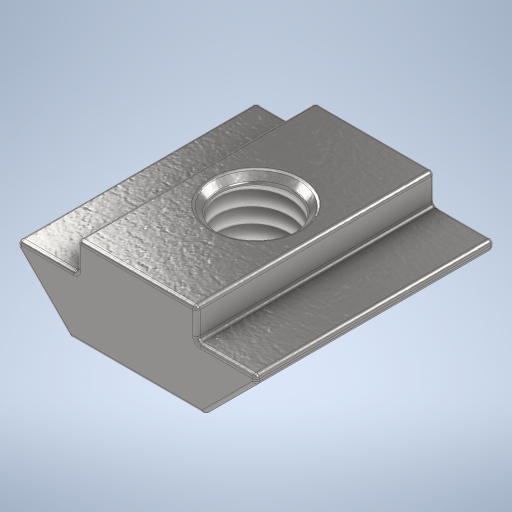
# Autodesk Inventor part: M6 T SLOT NUT 3030
Saved by Autodesk Inventor 2024 (Build 280153000, 153)
## iProperties
Created: 2024-12-02
Part Number: M6 T SLOT NUT 3030
Material: Steel, Galvanized
Document SubType Name: Modeling
Designer: Ishaan
Density: 7.85 g/cm^3
Appearance: Galvanized
Author: Ishaan
Autodesk Inventor part; units mm, degrees
ref_plane "YZ Plane" through (0, 0, 0) normal (1, 0, 0) x (0, 1, 0)
ref_plane "XZ Plane" through (0, 0, 0) normal (0, 1, 0) x (-1, 0, 0)
ref_plane "XY Plane" through (0, 0, 0) normal (0, 0, 1) x (1, 0, 0)
sketch "Sketch1" plane through (0, 0, 0) normal (0, 0, 1) x (1, 0, 0)
  line L0 (4, -3) -> (-4, -3)
  line L1 (-4, -3) -> (-4, 3)
  line L2 (-4, 3) -> (4, 3)
  line L3 (4, 3) -> (4, -3)
  line L4 (4, -3) -> (-4, 3) construction
  line L5 (-4, -3) -> (4, 3) construction
  line L6 (-8, 1) -> (8, 1)
  line L7 (8, 1) -> (8, -3)
  line L8 (8, -3) -> (-8, -3)
  line L9 (-8, -3) -> (-8, 1)
  point P0 (0, 0)
  point P1 (0, -3)
  point P2 (4, 1)
  point P3 (-4, 1)
  dimension "d0" = 2
  dimension "d1" = 4
  dimension "d2" = 16
  dimension "d3" = 8
  constraints: 20 end point, 4 midpoint, 4 parallel, 2 horizontal, 2 perpendicular
  measures "d0" distance between parallel lines of L2 L6
  measures "d1" distance of L8.end L6.start
  measures "d2" distance of L7.end L8.end
  measures "d3" distance of L1.end L2.end
extrude "Extrusion1" add sketch "Sketch1" along normal mid plane 16
chamfer "Chamfer1" distance 3.5 angle 45 2 edges at (-8, -3, 0) (8, -3, 0)
sketch "Sketch2" plane through (-4, 3, 8) normal (0, 1, 0) x (1, 0, 0)
  point P0 (4, 8)
hole "Hole1" at (0, 3, 0) direction (0, -1, 0) diameter 4.917 end through all thread size "M6x1" class "6H" standard "ANSI Metric M Profile"
chamfer "Chamfer2" distance 0.5 angle 45 2 edges at (0, 3, -2.4585) (0, -3, -2.4585)
fillet "Fillet1" radius 0.25 34 edges at (0, -3, 8) (8, 0.75, 8) (6.25, -1.25, 8) (4, 2, 8) (0, 3, 8) (-6.25, -1.25, 8) (-8, 0.75, 8) (-6, 1, 8) (-4, 2, 8) (6, 1, 8) (4, 2, -8) (0, -3, -8) (0, 3, -8) (-6.25, -1.25, -8) (-6, 1, -8) (-8, 0.75, -8) (6.25, -1.25, -8) (6, 1, -8) (8, 0.75, -8) (-4, 2, -8) (0, -2.5, -2.4585) (0, 3, -2.9585) (-8, 0.5, 0) (-4.5, -3, 0) (-4, 1, 0) (-4, 3, 0) (4.5, -3, 0) (4, 1, 0) (8, 1, 0) (8, 0.5, 0) (0, -3, -2.9585) (0, 2.5, -2.4585) (4, 3, 0) (-8, 1, 0)
body "Solid1"
